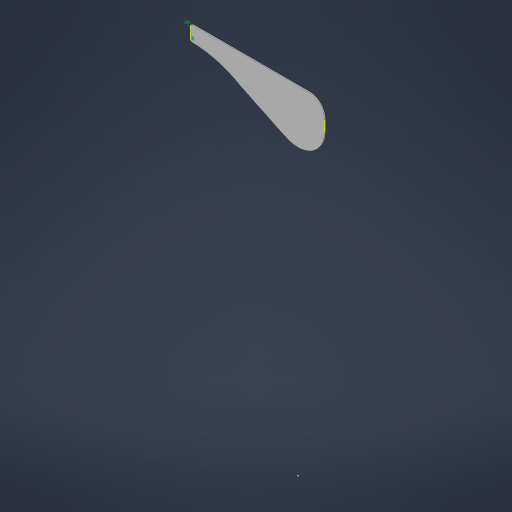
# Autodesk Inventor part: Better intake poly
Saved by Autodesk Inventor 2023.4 (Build 274418000, 418)
## iProperties
Created: 2023-12-16
Part Number: Better intake poly
Material: Generic
Document SubType Name: Modeling
Designer: diego
Density: 1 g/cm^3
Appearance: Default
Author: diego
Autodesk Inventor part; units mm, degrees
ref_plane "YZ Plane" through (0, 0, 0) normal (1, 0, 0) x (0, 1, 0)
ref_plane "XZ Plane" through (0, 0, 0) normal (0, 1, 0) x (-1, 0, 0)
ref_plane "XY Plane" through (0, 0, 0) normal (0, 0, 1) x (1, 0, 0)
sketch "Sketch1" plane through (0, 0, 0) normal (0, 0, 1) x (1, 0, 0)
  circle A0 centre (0, 0) radius 25.4
  line L0 (0, 25.4) -> (-203.2, 25.4)
  line L1 (-203.2, 25.4) -> (-203.2, -12.7)
  line L2 (25.4, 0) -> (203.2, 0) construction
  line L3 (203.2, 0) -> (203.2, -127) construction
  arc A1 (203.2, -127) -> (-203.2, -12.7) centre (-98.0265, -418.3887) ccw construction
  line L4 (-203.2, 25.4) -> (-203.2, -50.8) construction
  arc A2 (203.2, -222.1538) -> (-203.2, -12.7) centre (-125.6377, -361.1999) ccw
  line L5 (-203.2, 25.4) -> (-203.2, 36.3602)
  line L6 (25.4, 0) -> (25.4, 25.4)
  line L7 (25.4, 25.4) -> (0, 25.4)
  circle A3 centre (0, 549.5888) radius 46.99
  line L8 (0, 596.5788) -> (-190.5, 596.5788)
  line L9 (46.99, 549.5888) -> (46.99, 596.5788)
  line L10 (46.99, 596.5788) -> (0, 596.5788)
  line L11 (46.99, 596.5788) -> (224.79, 596.5788)
  line L12 (224.79, 596.5788) -> (224.79, 190.1788)
  line L13 (0, 596.5788) -> (-190.5, 596.5788) construction
  line L14 (-190.5, 596.5788) -> (-190.5, 558.4788) construction
  line L15 (-190.5, 596.5788) -> (-190.5, 558.4788)
  line L16 (-190.5, 596.5788) -> (0, 596.5788)
  line L17 (0, 596.5788) -> (-101.6, 596.5788)
  line L18 (-101.6, 596.5788) -> (-101.6, 545.7788)
  line L19 (-101.6, 545.7788) -> (-46.99, 545.7788)
  line L20 (224.79, 190.1788) -> (-334.01, 190.1788)
  line L21 (23.495, -36.812) -> (-174.1484, -525.1707)
  line L22 (203.2, -222.1538) -> (-203.2, -12.7)
  line L23 (224.79, 264.9183) -> (-394.0921, 264.9183)
  line L24 (224.79, 596.5788) -> (224.79, 393.3788)
  line L25 (224.79, 393.3788) -> (-334.01, 393.3788)
  line L26 (0, 502.5988) -> (0, 393.3788)
  arc A4 (-101.6, 545.7788) -> (-247.5257, 560.3429) centre (-190.5, 393.3788) ccw
  spline S0 degree 2 poles (-101.6, 545.7788) (2.3295, 495.7011) (-25.4, 510.0552) knots 0 0 0 1 1 1
  point P0 (-19.5605, 506.8635)
  point P1 (-190.5, 569.8128)
  dimension "d0" = 50.8
  dimension "d1" = 203.2
  dimension "d2" = 177.8
  dimension "d3" = 127
  dimension "d4" = 38.1
  dimension "d5" = 419.1
  dimension "d6" = 76.2
  dimension "d7" = 457.2
  dimension "d8" = 93.98
  dimension "d11" = 177.8
  dimension "d12" = 406.4
  dimension "d13" = 190.5
  dimension "d14" = 38.1
  dimension "d18" = 101.6
  dimension "d19" = 558.8
  dimension "d20" = 203.2
  dimension "d21" = 558.8
  constraints: 54 end point, 15 point on circle, 11 perpendicular, 6 point on line, 6 tangent, 5 centre point, 5 horizontal, 2 collinear, 2 vertical, 1 coincident, 1 midpoint, 3 other
  measures "d0" diameter of A0
  measures "d1" distance of L0.start L0.end
  measures "d2" distance of L2.start L2.end
  measures "d3" distance of L2.end L3.end
  measures "d4" distance of L0.end L1.end
  measures "d5" radius of A1
  measures "d6" distance of L0.end L4.end
  measures "d7" distance of L1.end L22.start
  measures "d8" diameter of A3
  measures "d11" distance of L9.end L11.end
  measures "d12" distance of L11.end L12.end
  measures "d13" distance of L8.end L8.start
  measures "d14" distance of L8.end L14.end
  measures "d18" distance of L8.start L17.end
  measures "d19" distance of L12.end L20.end
  measures "d20" distance of L11.end L24.end
  measures "d21" distance of L24.end L25.end
extrude "Extrusion2" add sketch "Sketch1" along normal blind 1.5875 contours A3 S0 | A3 L10 L9 | A3 S0 L18 L8 | S0 A3 | L18 A4 L15 L8
fillet "Fillet2" radius 28.575 1 edges at (46.99, 596.5788, 0.7937)
fillet "Fillet3" radius 3.175 1 edges at (-190.5, 596.5788, 0.7937)
fillet "Fillet4" radius 3.175 1 edges at (-190.5, 569.8128, 0.7937)
sketch "Sketch3" plane through (0, 0, 1.5875) normal (0, 0, 1) x (1, 0, 0)
  circle A0 centre (-186.1685, 576.5475) radius 2.54
  point P0 (0, 0)
  dimension "d27" = 5.08
  constraints: 1 centre point
  measures "d27" diameter of A0
sketch "Sketch4" plane through (0, 0, 1.5875) normal (0, 0, 1) x (1, 0, 0)
  line L0 (-190.5, 593.4038) -> (-190.5, 572.9597) projected
  line L1 (46.99, 549.5888) -> (46.99, 568.0038) projected
  point P0 (0, 0)
body "Solid2"
